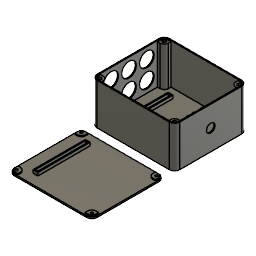
AC Box and Lid (Autodesk Fusion 360 design; units mm, degrees)
Autodesk Fusion 360 part; units mm, degrees
(part 1 of 2)
sketch "Sketch1" plane through (0, 0, 0) normal (0, 1, 0) x (1, 0, 0)
  line L0 (12.7, -101.6) -> (-165.1, -101.6)
  line L1 (-177.8, -88.9) -> (-177.8, 63.5)
  line L2 (-165.1, 76.2) -> (12.7, 76.2)
  line L3 (25.4, 63.5) -> (25.4, -88.9)
  arc A0 (-165.1, 76.2) -> (-177.8, 63.5) centre (-165.1, 63.5) ccw
  arc A1 (-177.8, -88.9) -> (-165.1, -101.6) centre (-165.1, -88.9) ccw
  arc A2 (25.4, 63.5) -> (12.7, 76.2) centre (12.7, 63.5) ccw
  arc A3 (12.7, -101.6) -> (25.4, -88.9) centre (12.7, -88.9) ccw
  line L4 (-158.75, 57.15) -> (-177.8, 57.15)
  line L5 (-177.8, 57.15) -> (-177.8, 76.2)
  line L6 (-177.8, 76.2) -> (-158.75, 76.2)
  line L7 (-158.75, 76.2) -> (-158.75, 57.15)
  line L8 (-164.275, 68.9844) -> (-168.275, 71.2938)
  line L9 (-168.275, 71.2938) -> (-172.275, 68.9844)
  line L10 (-172.275, 68.9844) -> (-172.275, 64.3656)
  line L11 (-172.275, 64.3656) -> (-168.275, 62.0562)
  line L12 (-168.275, 62.0562) -> (-164.275, 64.3656)
  line L13 (-164.275, 64.3656) -> (-164.275, 68.9844)
  line L14 (6.35, 76.2) -> (25.4, 76.2)
  line L15 (25.4, 57.15) -> (6.35, 57.15)
  line L16 (11.875, 68.9844) -> (11.875, 64.3656)
  line L17 (19.875, 64.3656) -> (19.875, 68.9844)
  line L18 (25.4, 76.2) -> (25.4, 57.15)
  line L19 (19.875, 68.9844) -> (15.875, 71.2938)
  line L20 (15.875, 71.2938) -> (11.875, 68.9844)
  line L21 (11.875, 64.3656) -> (15.875, 62.0562)
  line L22 (15.875, 62.0562) -> (19.875, 64.3656)
  line L23 (6.35, 57.15) -> (6.35, 76.2)
  line L24 (-177.8, -82.55) -> (-158.75, -82.55)
  line L25 (-158.75, -101.6) -> (-177.8, -101.6)
  line L26 (-172.275, -89.7656) -> (-172.275, -94.3844)
  line L27 (-164.275, -94.3844) -> (-164.275, -89.7656)
  line L28 (-158.75, -82.55) -> (-158.75, -101.6)
  line L29 (-164.275, -89.7656) -> (-168.275, -87.4562)
  line L30 (-168.275, -87.4562) -> (-172.275, -89.7656)
  line L31 (-172.275, -94.3844) -> (-168.275, -96.6938)
  line L32 (-168.275, -96.6938) -> (-164.275, -94.3844)
  line L33 (-177.8, -101.6) -> (-177.8, -82.55)
  line L34 (6.35, -82.55) -> (25.4, -82.55)
  line L35 (25.4, -101.6) -> (6.35, -101.6)
  line L36 (11.875, -89.7656) -> (11.875, -94.3844)
  line L37 (19.875, -94.3844) -> (19.875, -89.7656)
  line L38 (25.4, -82.55) -> (25.4, -101.6)
  line L39 (19.875, -89.7656) -> (15.875, -87.4562)
  line L40 (15.875, -87.4562) -> (11.875, -89.7656)
  line L41 (11.875, -94.3844) -> (15.875, -96.6938)
  line L42 (15.875, -96.6938) -> (19.875, -94.3844)
  line L43 (6.35, -101.6) -> (6.35, -82.55)
  circle A4 centre (-168.275, 66.675) radius 3.175
  circle A5 centre (-168.275, -92.075) radius 3.175
  circle A6 centre (15.875, -92.075) radius 3.175
  circle A7 centre (15.875, 66.675) radius 3.175
  point P0 (0, -101.6)
  point P1 (-177.8, -101.6)
  point P2 (25.4, 76.2)
  point P3 (-168.275, 66.675)
  point P4 (-6.35, 76.2)
  point P5 (-19.05, 63.5)
  point P6 (-6.35, 63.5)
  point P7 (15.875, 66.675)
  point P8 (-165.1, -82.55)
  point P9 (-177.8, -19.05)
  point P10 (-165.1, -95.25)
  point P11 (-168.275, -92.075)
  point P12 (-6.35, -6.35)
  point P13 (-19.05, -19.05)
  point P14 (-6.35, -19.05)
  point P15 (15.875, -92.075)
  dimension "d1" = 177.8
  dimension "d3" = 12.7
  dimension "d4" = 12.7
  dimension "d5" = 12.7
  dimension "d6" = 12.7
  dimension "d7" = 4
  dimension "d12" = 6.35
  dimension "d13" = 6.35
  dimension "d14" = 6.35
  dimension "d15" = 6.35
  dimension "d138" = 203.2
  dimension "d195" = 152.4
  constraint vertical L1
  constraint horizontal L2
  constraint vertical L3
  constraint tangent L1 A0
  constraint tangent L2 A0
  constraint coincident P1 L1
  constraint coincident P1 L0
  constraint tangent L1 A1
  constraint tangent L0 A1
  constraint coincident P2 L2
  constraint coincident P2 L3
  constraint tangent L2 A2
  constraint tangent L3 A2
  constraint tangent L3 A3
  constraint tangent L0 A3
  constraint horizontal L4
  constraint vertical L5
  constraint horizontal L6
  constraint vertical L7
  constraint coincident P3 A4.centre
  constraint coincident P11 A5.centre
  constraint coincident P15 A6.centre
  constraint coincident P7 A7.centre
  measures "d1" distance of P0 L25.end
  measures "d3" radius of A0
  measures "d4" radius of A1
  measures "d5" radius of A2
  measures "d6" radius of A3
  measures "d7" distance of P3 L13
  measures "d12" diameter of A4
  measures "d13" diameter of A5
  measures "d14" diameter of A6
  measures "d15" diameter of A7
  measures "d138" distance of L1 L3
  measures "d195" distance of L1.end L1.start
  measures "d385" diameter of L27.end
extrude "Extrude1" add sketch "Sketch1" along normal blind 101.6 contours L0 L3 A3 L34 L35 L38 L43 | L0 L1 L2 L3 L4 L7 L15 L23 L24 L28 L34 L43 | L0 L1 A1 L24 L25 L28 L33 | L2 L3 A2 L14 L15 L18 L23 | L1 L2 A0 L4 L5 L6 L7 | L8 L9 L10 L11 L12 L13 | L16 L17 L19 L20 L21 L22 | L26 L27 L29 L30 L31 L32 | L36 L37 L39 L40 L41 L42 | A4 | A5 | A6 | A7 makes body 1
shell "Shell1" thickness 2.54 removed faces 1 at (-103.7167, 101.6, -16.9333) on bodies 1
extrude "Extrude2" add sketch "Sketch1" along normal blind 99.06 contours L0 L3 A3 L34 L35 L38 L43 | L0 L1 A1 L24 L25 L28 L33 | L2 L3 A2 L14 L15 L18 L23 | L1 L2 A0 L4 L5 L6 L7 bodies 1
extrude "Extrude3" add sketch "Sketch1" along normal blind 93.98 contours L8 L9 L10 L11 L12 L13 | L16 L17 L19 L20 L21 L22 | L26 L27 L29 L30 L31 L32 | L36 L37 L39 L40 L41 L42 bodies 1
fillet "Fillet1" radius 10.16 4 edges at (-158.75, 50.8, -57.15) (-158.75, 50.8, 82.55) (6.35, 50.8, -57.15) (6.35, 50.8, 82.55) on bodies 1
sketch "Sketch3" plane through (0, 0, 0) normal (0, 1, 0) x (1, 0, 0)
  line L0 (-165.1, -127) -> (12.7, -127)
  line L1 (25.4, -139.7) -> (25.4, -292.1)
  line L2 (12.7, -304.8) -> (-165.1, -304.8)
  line L3 (-177.8, -292.1) -> (-177.8, -139.7)
  arc A0 (-165.1, -127) -> (-177.8, -139.7) centre (-165.1, -139.7) ccw
  arc A1 (25.4, -139.7) -> (12.7, -127) centre (12.7, -139.7) ccw
  arc A2 (-177.8, -292.1) -> (-165.1, -304.8) centre (-165.1, -292.1) ccw
  arc A3 (12.7, -304.8) -> (25.4, -292.1) centre (12.7, -292.1) ccw
  line L4 (-168.91, -146.05) -> (-177.8, -146.05)
  line L5 (-177.8, -146.05) -> (-177.8, -127)
  line L6 (-177.8, -127) -> (-158.75, -127)
  line L7 (-158.75, -127) -> (-158.75, -135.89)
  circle A4 centre (-168.275, -136.525) radius 3
  line L8 (25.4, -285.75) -> (16.51, -285.75)
  line L9 (6.35, -295.91) -> (6.35, -304.8)
  line L10 (6.35, -304.8) -> (25.4, -304.8)
  line L11 (25.4, -304.8) -> (25.4, -285.75)
  circle A5 centre (15.875, -295.275) radius 3
  circle A6 centre (15.875, -136.525) radius 3
  circle A7 centre (-168.275, -295.275) radius 3
  line L12 (-177.8, -304.8) -> (-158.75, -304.8)
  line L13 (-158.75, -304.8) -> (-158.75, -295.91)
  line L14 (-168.91, -285.75) -> (-177.8, -285.75)
  line L15 (-177.8, -285.75) -> (-177.8, -304.8)
  line L16 (16.51, -146.05) -> (25.4, -146.05)
  line L17 (25.4, -146.05) -> (25.4, -127)
  line L18 (25.4, -127) -> (6.35, -127)
  line L19 (6.35, -127) -> (6.35, -135.89)
  arc A8 (-168.91, -146.05) -> (-158.75, -135.89) centre (-168.91, -135.89) ccw
  arc A9 (-158.75, -295.91) -> (-168.91, -285.75) centre (-168.91, -295.91) ccw
  arc A10 (6.35, -135.89) -> (16.51, -146.05) centre (16.51, -135.89) ccw
  arc A11 (16.51, -285.75) -> (6.35, -295.91) centre (16.51, -295.91) ccw
  arc A12 (-165.1, -129.54) -> (-175.26, -139.7) centre (-165.1, -139.7) ccw
  line L20 (-175.26, -292.1) -> (-175.26, -139.7)
  arc A13 (-175.26, -292.1) -> (-165.1, -302.26) centre (-165.1, -292.1) ccw
  line L21 (12.7, -302.26) -> (-165.1, -302.26)
  arc A14 (12.7, -302.26) -> (22.86, -292.1) centre (12.7, -292.1) ccw
  line L22 (22.86, -139.7) -> (22.86, -292.1)
  arc A15 (22.86, -139.7) -> (12.7, -129.54) centre (12.7, -139.7) ccw
  line L23 (-165.1, -129.54) -> (12.7, -129.54)
  line L24 (6.35, -129.54) -> (3.81, -129.54)
  circle A16 centre (-168.275, -136.525) radius 5
  circle A17 centre (-168.275, -295.275) radius 5
  circle A18 centre (15.875, -295.275) radius 5
  circle A19 centre (15.875, -136.525) radius 5
  dimension "d28" = 12.7
  dimension "d29" = 12.7
  dimension "d30" = 12.7
  dimension "d31" = 12.7
  dimension "d32" = 6
  dimension "d34" = 6
  dimension "d35" = 6
  dimension "d36" = 6
  dimension "d39" = 19.05
  dimension "d40" = 10.16
  dimension "d41" = 10.16
  dimension "d42" = 10.16
  dimension "d43" = 10.16
  dimension "d44" = 2.54
  dimension "d68" = 10
  dimension "d69" = 10
  dimension "d70" = 10
  dimension "d71" = 10
  dimension "d139" = 198.12
  dimension "d196" = 152.4
  constraint horizontal L0
  constraint vertical L1
  constraint horizontal L2
  constraint vertical L3
  constraint tangent L0 A0
  constraint tangent L3 A0
  constraint tangent L0 A1
  constraint tangent L1 A1
  constraint tangent L3 A2
  constraint tangent L2 A2
  constraint tangent L1 A3
  constraint tangent L2 A3
  constraint horizontal L4
  constraint vertical L5
  constraint horizontal L6
  constraint vertical L7
  constraint horizontal L8
  constraint vertical L9
  constraint horizontal L10
  constraint vertical L11
  constraint horizontal L12
  constraint vertical L13
  constraint horizontal L14
  constraint vertical L15
  constraint horizontal L16
  constraint vertical L17
  constraint horizontal L18
  constraint vertical L19
  constraint tangent L4 A8
  constraint tangent L7 A8
  constraint tangent L13 A9
  constraint tangent L14 A9
  constraint tangent L16 A10
  constraint tangent L19 A10
  constraint tangent L8 A11
  constraint tangent L9 A11
  constraint horizontal L24
  constraint coincident L23 L24.start
  constraint coincident L19 L24.start
  constraint concentric A4 A16
  constraint concentric A7 A17
  constraint concentric A5 A18
  constraint concentric A6 A19
  measures "d28" radius of A0
  measures "d29" radius of A1
  measures "d30" radius of A2
  measures "d31" radius of A3
  measures "d32" diameter of A4
  measures "d34" diameter of A5
  measures "d35" diameter of A6
  measures "d36" diameter of A7
  measures "d39" distance of L12.start L14.end
  measures "d40" radius of A8
  measures "d41" radius of A9
  measures "d42" radius of A10
  measures "d43" radius of A11
  measures "d68" diameter of A16
  measures "d69" diameter of A17
  measures "d70" diameter of A18
  measures "d71" diameter of A19
  measures "d139" distance of L20 L22
  measures "d196" distance of L3.end L3.start
extrude "Extrude5" add sketch "Sketch3" along normal blind 3.81 separate body contours L0 L3 A0 L4 L5 L6 L7 A12 L20 L23 | L0 L7 L19 L23 L24 | L0 L1 A1 L16 L17 L18 L19 L22 A15 L23 | L4 L7 L8 L9 L13 L14 L16 L19 A8 A9 A10 A11 L20 L21 L22 L23 L24 | L4 L7 A8 A12 L20 L23 | L3 L4 L14 L20 | L16 L19 A10 L22 A15 L23 | L2 L3 A2 L12 L13 L14 L15 L20 A13 L21 | L13 L14 A9 L20 A13 L21 | L1 L8 L16 L22 | L1 L2 A3 L8 L9 L10 L11 L21 A14 L22 | L2 L9 L13 L21 | L8 L9 A11 L21 A14 L22 | A16 | A17 | A18 | A19 makes body 2
extrude "Extrude6" add sketch "Sketch3" along normal blind 6.35 contours L4 L7 A8 A12 L20 L23 | L16 L19 A10 L22 A15 L23 | L13 L14 A9 L20 A13 L21 | L8 L9 A11 L21 A14 L22 | A16 | A17 | A18 | A19 bodies 2
chamfer "Chamfer1" distance 2.032 angle 45 4 edges at (13.078, 0, 135.4402) (13.078, 0, 294.1902) (-171.072, 0, 135.4402) (-171.072, 0, 294.1902) on bodies 2
sketch "Sketch10" plane through (-175.26, 0, 0) normal (1, 0, 0) x (0, 0, -1)
  line L0 (57.15, 2.54) -> (57.15, 99.06)
  line L1 (57.15, 99.06) -> (63.5, 99.06)
  line L2 (63.5, 99.06) -> (63.5, 101.6)
  line L3 (63.5, 101.6) -> (-88.9, 101.6)
  line L4 (-88.9, 101.6) -> (-88.9, 99.06)
  line L5 (-88.9, 99.06) -> (-82.55, 99.06)
  line L6 (-82.55, 99.06) -> (-82.55, 2.54)
  line L7 (-82.55, 2.54) -> (57.15, 2.54)
  line L8 (-82.55, 2.54) -> (-82.55, 101.6) construction
  line L9 (-82.55, 101.6) -> (-74.2569, 101.6) construction
  line L10 (-74.2569, 101.6) -> (-74.2569, 92.2528) construction
  line L11 (-74.2569, 92.2528) -> (-82.55, 92.2528) construction
  line L12 (-82.55, 92.2528) -> (-82.55, 101.6) construction
  line L13 (57.15, 101.6) -> (31.1023, 101.6) construction
  line L14 (31.1023, 101.6) -> (31.1023, 74.4982) construction
  line L15 (31.1023, 74.4982) -> (57.15, 74.4982) construction
  line L16 (57.15, 74.4982) -> (57.15, 101.6) construction
  circle A0 centre (31.1023, 74.4982) radius 17.7546
  line L17 (-82.55, 101.6) -> (-56.5023, 101.6) construction
  line L18 (-56.5023, 101.6) -> (-56.5023, 74.4982) construction
  line L19 (-56.5023, 74.4982) -> (-82.55, 74.4982) construction
  line L20 (-82.55, 74.4982) -> (-82.55, 101.6) construction
  line L21 (-56.5023, 2.54) -> (-56.5023, 29.6418) construction
  line L22 (-56.5023, 74.4982) -> (31.1023, 74.4982) construction
  circle A1 centre (-12.7, 74.4982) radius 17.7546
  circle A2 centre (-56.5023, 74.4982) radius 17.7546
  circle A3 centre (31.1023, 29.6418) radius 17.7546
  circle A4 centre (-12.7, 29.6418) radius 17.7546
  circle A5 centre (-56.5023, 29.6418) radius 17.7546
  line L23 (-38.7477, 74.4982) -> (-38.7477, 2.54) construction
  line L24 (-74.2569, 74.4982) -> (-74.2569, 2.54) construction
  line L25 (-30.4546, 74.4982) -> (-30.4546, 2.54) construction
  line L26 (5.0546, 74.4982) -> (5.0546, 2.54) construction
  line L27 (13.3477, 74.4982) -> (13.3477, 2.54) construction
  line L28 (48.8569, 74.4982) -> (48.8569, 2.54) construction
  line L29 (-39.0023, 91.9982) -> (-39.0023, 56.9982)
  line L30 (-56.5023, 74.4982) -> (-39.0023, 74.4982) construction
  line L31 (-56.5023, 91.9982) -> (-56.5023, 56.9982) construction
  circle A6 centre (-50.7316, 77.9802) radius 3.7
  circle A7 centre (-62.3334, 77.8956) radius 3.7
  line L32 (-39.0023, 74.4982) -> (-39.0023, 91.9982) construction
  line L33 (-39.0023, 56.9982) -> (-74.0023, 56.9982)
  circle A8 centre (-50.3617, 86.7403) radius 1.25
  line L34 (-39.0023, 56.9982) -> (-39.0023, 91.9982) construction
  circle A9 centre (-56.5023, 74.4982) radius 17.5
  circle A10 centre (-65.2414, 63.5652) radius 1.25
  circle A11 centre (-59.9313, 63.1667) radius 3
  line L35 (-74.0023, 91.9982) -> (-39.0023, 91.9982)
  line L36 (-74.0023, 74.4982) -> (-39.0023, 74.4982) construction
  line L37 (-74.0023, 56.9982) -> (-74.0023, 91.9982)
  line L38 (-39.0023, 91.9982) -> (-56.5023, 91.9982) construction
  line L39 (-56.5023, 91.9982) -> (-56.5023, 74.4982) construction
  line L40 (4.8, 91.9982) -> (4.8, 56.9982)
  line L41 (-12.7, 74.4982) -> (4.8, 74.4982) construction
  line L42 (-12.7, 91.9982) -> (-12.7, 56.9982) construction
  circle A12 centre (-6.9293, 77.9802) radius 3.7
  circle A13 centre (-18.5311, 77.8956) radius 3.7
  line L43 (4.8, 74.4982) -> (4.8, 91.9982) construction
  line L44 (4.8, 56.9982) -> (-30.2, 56.9982)
  circle A14 centre (-6.5594, 86.7403) radius 1.25
  line L45 (4.8, 56.9982) -> (4.8, 91.9982) construction
  circle A15 centre (-12.7, 74.4982) radius 17.5
  circle A16 centre (-21.4391, 63.5652) radius 1.25
  circle A17 centre (-16.129, 63.1667) radius 3
  line L46 (-30.2, 91.9982) -> (4.8, 91.9982)
  line L47 (-30.2, 74.4982) -> (4.8, 74.4982) construction
  line L48 (-30.2, 56.9982) -> (-30.2, 91.9982)
  line L49 (4.8, 91.9982) -> (-12.7, 91.9982) construction
  line L50 (-12.7, 91.9982) -> (-12.7, 74.4982) construction
  line L51 (-74.0023, 29.6418) -> (-39.0023, 29.6418) construction
  line L52 (-56.5023, 29.6418) -> (-39.0023, 29.6418) construction
  circle A18 centre (-56.5023, 29.6418) radius 17.5
  line L53 (-39.0023, 29.6418) -> (-39.0023, 47.1418) construction
  circle A19 centre (-65.2414, 18.7088) radius 1.25
  line L54 (-56.5023, 47.1418) -> (-56.5023, 29.6418) construction
  line L55 (-39.0023, 47.1418) -> (-39.0023, 12.1418)
  circle A20 centre (-50.3617, 41.8839) radius 1.25
  line L56 (-39.0023, 12.1418) -> (-74.0023, 12.1418)
  line L57 (-74.0023, 12.1418) -> (-74.0023, 47.1418)
  circle A21 centre (-59.9313, 18.3103) radius 3
  line L58 (-39.0023, 47.1418) -> (-56.5023, 47.1418) construction
  line L59 (-74.0023, 47.1418) -> (-39.0023, 47.1418)
  line L60 (-56.5023, 47.1418) -> (-56.5023, 12.1418) construction
  circle A22 centre (-50.7316, 33.1238) radius 3.7
  circle A23 centre (-62.3334, 33.0392) radius 3.7
  line L61 (-39.0023, 12.1418) -> (-39.0023, 47.1418) construction
  line L62 (-30.2, 29.6418) -> (4.8, 29.6418) construction
  line L63 (-30.2, 47.1418) -> (4.8, 47.1418)
  circle A24 centre (-12.7, 29.6418) radius 17.5
  line L64 (-12.7, 29.6418) -> (4.8, 29.6418) construction
  circle A25 centre (-16.129, 18.3103) radius 3
  line L65 (4.8, 47.1418) -> (-12.7, 47.1418) construction
  line L66 (-12.7, 47.1418) -> (-12.7, 29.6418) construction
  circle A26 centre (-18.5311, 33.0392) radius 3.7
  line L67 (4.8, 47.1418) -> (4.8, 12.1418)
  line L68 (-12.7, 47.1418) -> (-12.7, 12.1418) construction
  line L69 (4.8, 29.6418) -> (4.8, 47.1418) construction
  line L70 (4.8, 12.1418) -> (4.8, 47.1418) construction
  circle A27 centre (-6.5594, 41.8839) radius 1.25
  line L71 (4.8, 12.1418) -> (-30.2, 12.1418)
  circle A28 centre (-6.9293, 33.1238) radius 3.7
  circle A29 centre (-21.4391, 18.7088) radius 1.25
  line L72 (-30.2, 12.1418) -> (-30.2, 47.1418)
  line L73 (13.6023, 29.6418) -> (48.6023, 29.6418) construction
  line L74 (13.6023, 47.1418) -> (48.6023, 47.1418)
  circle A30 centre (31.1023, 29.6418) radius 17.5
  line L75 (31.1023, 29.6418) -> (48.6023, 29.6418) construction
  circle A31 centre (27.6733, 18.3103) radius 3
  line L76 (48.6023, 47.1418) -> (31.1023, 47.1418) construction
  line L77 (31.1023, 47.1418) -> (31.1023, 29.6418) construction
  circle A32 centre (25.2712, 33.0392) radius 3.7
  line L78 (48.6023, 47.1418) -> (48.6023, 12.1418)
  line L79 (31.1023, 47.1418) -> (31.1023, 12.1418) construction
  line L80 (48.6023, 29.6418) -> (48.6023, 47.1418) construction
  line L81 (48.6023, 12.1418) -> (48.6023, 47.1418) construction
  circle A33 centre (37.2429, 41.8839) radius 1.25
  line L82 (48.6023, 12.1418) -> (13.6023, 12.1418)
  circle A34 centre (36.873, 33.1238) radius 3.7
  circle A35 centre (22.3632, 18.7088) radius 1.25
  line L83 (13.6023, 12.1418) -> (13.6023, 47.1418)
  line L84 (13.6023, 74.4982) -> (48.6023, 74.4982) construction
  line L85 (13.6023, 91.9982) -> (48.6023, 91.9982)
  circle A36 centre (31.1023, 74.4982) radius 17.5
  line L86 (31.1023, 74.4982) -> (48.6023, 74.4982) construction
  circle A37 centre (27.6733, 63.1667) radius 3
  line L87 (48.6023, 91.9982) -> (31.1023, 91.9982) construction
  line L88 (31.1023, 91.9982) -> (31.1023, 74.4982) construction
  circle A38 centre (25.2712, 77.8956) radius 3.7
  line L89 (48.6023, 91.9982) -> (48.6023, 56.9982)
  line L90 (31.1023, 91.9982) -> (31.1023, 56.9982) construction
  line L91 (48.6023, 74.4982) -> (48.6023, 91.9982) construction
  line L92 (48.6023, 56.9982) -> (48.6023, 91.9982) construction
  circle A39 centre (37.2429, 86.7403) radius 1.25
  line L93 (48.6023, 56.9982) -> (13.6023, 56.9982)
  circle A40 centre (36.873, 77.9802) radius 3.7
  circle A41 centre (22.3632, 63.5652) radius 1.25
  line L94 (13.6023, 56.9982) -> (13.6023, 91.9982)
  line L95 (-74.0023, 91.9982) -> (-74.0161, 101.6) construction
  line L96 (-74.0161, 101.6) -> (48.6023, 101.6)
  line L97 (48.6023, 101.6) -> (48.6023, 2.54)
  line L98 (48.6023, 2.54) -> (-74.0161, 2.54)
  line L99 (-74.0161, 2.54) -> (-74.0161, 101.6)
  point P0 (-56.5023, 131.8455)
  point P1 (-56.5023, 74.4982)
  point P2 (-50.3617, 86.7403)
  point P3 (-56.5023, 131.8455)
  point P4 (-12.7, 154.7055)
  point P5 (-12.7, 74.4982)
  point P6 (-6.5594, 86.7403)
  point P7 (9.303, 164.289)
  point P8 (-12.7, 154.7055)
  point P9 (9.303, 164.289)
  point P10 (-50.3617, 41.8839)
  point P11 (-56.5023, 29.6418)
  point P12 (-56.5023, 154.7055)
  point P13 (-56.5023, 154.7055)
  point P14 (9.303, 164.289)
  point P15 (9.303, 164.289)
  point P16 (-12.7, 29.6418)
  point P17 (-12.7, 154.7055)
  point P18 (-6.5594, 41.8839)
  point P19 (-12.7, 154.7055)
  point P20 (9.303, 164.289)
  point P21 (9.303, 164.289)
  point P22 (31.1023, 29.6418)
  point P23 (31.1023, 154.7055)
  point P24 (37.2429, 41.8839)
  point P25 (31.1023, 154.7055)
  point P26 (9.303, 164.289)
  point P27 (9.303, 164.289)
  point P28 (31.1023, 74.4982)
  point P29 (31.1023, 154.7055)
  point P30 (37.2429, 86.7403)
  point P31 (31.1023, 154.7055)
  dimension "d199" = 8.2931
  dimension "d200" = 9.3472
  dimension "d201" = 26.0477
  dimension "d202" = 27.1018
  dimension "d203" = 35.5092
  dimension "d204" = 26.0477
  dimension "d205" = 27.1018
  dimension "d206" = 27.1018
  dimension "d207" = 87.6046
  dimension "d208" = 44.8564
  dimension "d211" = -87.6046
  dimension "d212" = -44.8564
  dimension "d271" = 2.5
  dimension "d272" = 35
  dimension "d273" = 2.5
  dimension "d274" = 7.4
  dimension "d275" = 7.4
  dimension "d276" = 6
  dimension "d277" = 12.2421
  dimension "d278" = 6.1406
  dimension "d279" = 5.7707
  dimension "d280" = 3.3974
  dimension "d281" = 5.8311
  dimension "d282" = 11.3315
  dimension "d283" = 3.482
  dimension "d284" = 8.7391
  dimension "d285" = 10.933
  dimension "d286" = 3.429
  dimension "d289" = 35
  dimension "d290" = 2.5
  dimension "d291" = 35
  dimension "d292" = 2.5
  dimension "d293" = 7.4
  dimension "d294" = 7.4
  dimension "d295" = 6
  dimension "d296" = 12.2421
  dimension "d297" = 6.1406
  dimension "d298" = 5.7707
  dimension "d299" = 3.3974
  dimension "d300" = 5.8311
  dimension "d301" = 11.3315
  dimension "d302" = 3.482
  dimension "d303" = 8.7391
  dimension "d304" = 10.933
  dimension "d305" = 3.429
  dimension "d306" = 35
  dimension "d307" = 2.5
  dimension "d308" = 35
  dimension "d309" = 2.5
  dimension "d310" = 7.4
  dimension "d311" = 7.4
  dimension "d312" = 6
  dimension "d313" = 12.2421
  dimension "d314" = 6.1406
  dimension "d315" = 5.7707
  dimension "d316" = 3.3974
  dimension "d317" = 5.8311
  dimension "d318" = 11.3315
  dimension "d319" = 3.482
  dimension "d320" = 8.7391
  dimension "d321" = 10.933
  dimension "d322" = 3.429
  dimension "d323" = 35
  dimension "d324" = 2.5
  dimension "d325" = 35
  dimension "d326" = 2.5
  dimension "d327" = 7.4
  dimension "d328" = 7.4
  dimension "d329" = 6
  dimension "d330" = 12.2421
  dimension "d331" = 6.1406
  dimension "d332" = 5.7707
  dimension "d333" = 3.3974
  dimension "d334" = 5.8311
  dimension "d335" = 11.3315
  dimension "d336" = 3.482
  dimension "d337" = 8.7391
  dimension "d338" = 10.933
  dimension "d339" = 3.429
  dimension "d340" = 35
  dimension "d341" = 2.5
  dimension "d342" = 35
  dimension "d343" = 2.5
  dimension "d344" = 7.4
  dimension "d345" = 7.4
  dimension "d346" = 6
  dimension "d347" = 12.2421
  dimension "d348" = 6.1406
  dimension "d349" = 5.7707
  dimension "d350" = 3.3974
  dimension "d351" = 5.8311
  dimension "d352" = 11.3315
  dimension "d353" = 3.482
  dimension "d354" = 8.7391
  dimension "d355" = 10.933
  dimension "d356" = 3.429
  dimension "d357" = 35
  dimension "d358" = 2.5
  dimension "d359" = 35
  dimension "d360" = 2.5
  dimension "d361" = 7.4
  dimension "d362" = 7.4
  dimension "d363" = 6
  dimension "d364" = 12.2421
  dimension "d365" = 6.1406
  dimension "d366" = 5.7707
  dimension "d367" = 3.3974
  dimension "d368" = 5.8311
  dimension "d369" = 11.3315
  dimension "d370" = 3.482
  dimension "d371" = 8.7391
  dimension "d372" = 10.933
  dimension "d373" = 3.429
  dimension "d374" = 35
  constraint coincident L6.end L7.start
  constraint coincident L3 L8.end
  constraint perpendicular L3 L8
  constraint horizontal L9
  constraint vertical L10
  constraint horizontal L11
  constraint vertical L12
  constraint horizontal L13
  constraint vertical L14
  constraint horizontal L15
  constraint vertical L16
  constraint coincident L3 L13.start
  constraint coincident P28 L14.end
  constraint horizontal L17
  constraint vertical L18
  constraint horizontal L19
  constraint vertical L20
  constraint coincident L7 L21.start
  constraint perpendicular L7 L21
  constraint coincident A2 L23.start
  constraint coincident L22 L23.start
  constraint coincident L7 L23.end
  constraint tangent A2 L23
  constraint coincident L19 L24.start
  constraint coincident A2 L24.start
  constraint coincident L7 L24.end
  constraint tangent A2 L24
  constraint coincident A1 L25.start
  constraint coincident L22 L25.start
  constraint coincident L7 L25.end
  constraint tangent A1 L25
  constraint coincident L22 L26.start
  constraint coincident A1 L26.start
  constraint coincident L7 L26.end
  constraint tangent A1 L26
  constraint coincident A0 L27.start
  constraint coincident L22 L27.start
  constraint coincident L7 L27.end
  constraint tangent A0 L27
  constraint coincident A0 L28.start
  constraint coincident L15 L28.start
  constraint coincident L7 L28.end
  constraint tangent A0 L28
  constraint coincident P2 A8.centre
  constraint midpoint P1 L36
  constraint coincident P1 L18.end
  constraint coincident L30.end A9
  constraint horizontal L36
  constraint perpendicular L30 L32
  constraint parallel L30 L38
  constraint parallel L32 L39
  constraint parallel L30 L36
  constraint midpoint L30.end L34
  constraint perpendicular L29 L33
  constraint parallel L29 L37
  constraint parallel L33 L35
  constraint midpoint L31.end L33
  constraint perpendicular L31 L33
  constraint coincident P3 L31
  constraint coincident P3 P0
  constraint coincident P6 A14.centre
  constraint midpoint P5 L47
  constraint coincident P5 A1.centre
  constraint coincident L41.end A15
  constraint horizontal L47
  constraint perpendicular L41 L43
  constraint parallel L41 L49
  constraint parallel L43 L50
  constraint parallel L41 L47
  constraint midpoint L41.end L45
  constraint perpendicular L40 L44
  constraint parallel L40 L48
  constraint parallel L44 L46
  constraint midpoint L42.end L44
  constraint perpendicular L42 L44
  constraint coincident P19 L42
  constraint coincident P19 P17
  constraint coincident P10 A20.centre
  constraint midpoint P11 L51
  constraint coincident P11 L21.end
  constraint coincident L51.end A18
  constraint horizontal L51
  constraint perpendicular L52 L53
  constraint parallel L52 L58
  constraint parallel L53 L54
  constraint parallel L51 L52
  constraint midpoint L51.end L61
  constraint perpendicular L55 L56
  constraint parallel L55 L57
  constraint parallel L56 L59
  constraint midpoint L60.end L56
  constraint perpendicular L56 L60
  constraint coincident P13 L60
  constraint coincident P13 P12
  constraint coincident P18 A27.centre
  constraint midpoint P16 L62
  constraint coincident P16 A4.centre
  constraint coincident L62.end A24
  constraint horizontal L62
  constraint perpendicular L64 L69
  constraint parallel L64 L65
  constraint parallel L66 L69
  constraint parallel L62 L64
  constraint midpoint L62.end L70
  constraint perpendicular L67 L71
  constraint parallel L67 L72
  constraint parallel L63 L71
  constraint midpoint L68.end L71
  constraint perpendicular L68 L71
  constraint coincident P19 L68
  constraint coincident P24 A33.centre
  constraint midpoint P22 L73
  constraint coincident P22 A3.centre
  constraint coincident L73.end A30
  constraint horizontal L73
  constraint perpendicular L75 L80
  constraint parallel L75 L76
  constraint parallel L77 L80
  constraint parallel L73 L75
  constraint midpoint L73.end L81
  constraint perpendicular L78 L82
  constraint parallel L78 L83
  constraint parallel L74 L82
  constraint midpoint L79.end L82
  constraint perpendicular L79 L82
  constraint coincident P31 L79
  constraint coincident P31 P29
  constraint coincident P30 A39.centre
  constraint midpoint P28 L84
  constraint coincident L84.end A36
  constraint horizontal L84
  constraint perpendicular L86 L91
  constraint parallel L86 L87
  constraint parallel L88 L91
  constraint parallel L84 L86
  constraint midpoint L84.end L92
  constraint perpendicular L89 L93
  constraint parallel L89 L94
  constraint parallel L85 L93
  constraint midpoint L90.end L93
  constraint perpendicular L90 L93
  constraint coincident P31 L90
  constraint coincident L17 L95.end
  constraint horizontal L96
  constraint vertical L97
  constraint horizontal L98
  constraint vertical L99
  constraint coincident L7 L97.end
  measures "d199" distance of L8.end L9.end
  measures "d200" distance of L8.end L11.end
  measures "d201" distance of L13.start L13.end
  measures "d202" distance of L13.start L15.end
  measures "d203" diameter of A0
  measures "d204" distance of L8.end L17.end
  measures "d205" distance of L8.end L19.end
  measures "d206" distance of L21.start P11
  measures "d207" distance of P28 P1
  measures "d208" distance of P1 P11
  measures "d271" diameter of A8
  measures "d272" diameter of A9
  measures "d273" diameter of A10
  measures "d274" diameter of A6
  measures "d275" diameter of A7
  measures "d276" diameter of A11
  measures "d277" vertical distance of P2 P1
  measures "d278" horizontal distance of P2 P1
  measures "d279" horizontal distance of P1 A6.centre
  measures "d280" vertical distance of A7.centre P1
  measures "d281" horizontal distance of A7.centre P1
  measures "d282" vertical distance of A11.centre P1
  measures "d283" vertical distance of P1 A6.centre
  measures "d284" horizontal distance of A10.centre P1
  measures "d285" vertical distance of A10.centre P1
  measures "d286" horizontal distance of A11.centre P1
  measures "d289" distance of L29.start L29.end
  measures "d290" diameter of A14
  measures "d291" diameter of A15
  measures "d292" diameter of A16
  measures "d293" diameter of A12
  measures "d294" diameter of A13
  measures "d295" diameter of A17
  measures "d296" vertical distance of P6 P5
  measures "d297" horizontal distance of P6 P5
  measures "d298" horizontal distance of P5 A12.centre
  measures "d299" vertical distance of A13.centre P5
  measures "d300" horizontal distance of A13.centre P5
  measures "d301" vertical distance of A17.centre P5
  measures "d302" vertical distance of P5 A12.centre
  measures "d303" horizontal distance of A16.centre P5
  measures "d304" vertical distance of A16.centre P5
  measures "d305" horizontal distance of A17.centre P5
  measures "d306" distance of L40.start L40.end
  measures "d307" diameter of A20
  measures "d308" diameter of A18
  measures "d309" diameter of A19
  measures "d310" diameter of A22
  measures "d311" diameter of A23
  measures "d312" diameter of A21
  measures "d313" vertical distance of P11 P10
  measures "d314" horizontal distance of P11 P10
  measures "d315" horizontal distance of A22.centre P11
  measures "d316" vertical distance of A23.centre P11
  measures "d317" horizontal distance of A23.centre P11
  measures "d318" vertical distance of A21.centre P11
  measures "d319" vertical distance of A22.centre P11
  measures "d320" horizontal distance of A19.centre P11
  measures "d321" vertical distance of A19.centre P11
  measures "d322" horizontal distance of A21.centre P11
  measures "d323" distance of L53.end L55.end
  measures "d324" diameter of A27
  measures "d325" diameter of A24
  measures "d326" diameter of A29
  measures "d327" diameter of A28
  measures "d328" diameter of A26
  measures "d329" diameter of A25
  measures "d330" vertical distance of P16 P18
  measures "d331" horizontal distance of P16 P18
  measures "d332" horizontal distance of P16 A28.centre
  measures "d333" vertical distance of A26.centre P16
  measures "d334" horizontal distance of A26.centre P16
  measures "d335" vertical distance of A25.centre P16
  measures "d336" vertical distance of P16 A28.centre
  measures "d337" horizontal distance of A29.centre P16
  measures "d338" vertical distance of A29.centre P16
  measures "d339" horizontal distance of A25.centre P16
  measures "d340" distance of L63.end L67.end
  measures "d341" diameter of A33
  measures "d342" diameter of A30
  measures "d343" diameter of A35
  measures "d344" diameter of A34
  measures "d345" diameter of A32
  measures "d346" diameter of A31
  measures "d347" vertical distance of P22 P24
  measures "d348" horizontal distance of P22 P24
  measures "d349" horizontal distance of P22 A34.centre
  measures "d350" vertical distance of A32.centre P22
  measures "d351" horizontal distance of A32.centre P22
  measures "d352" vertical distance of A31.centre P22
  measures "d353" vertical distance of P22 A34.centre
  measures "d354" horizontal distance of A35.centre P22
  measures "d355" vertical distance of A35.centre P22
  measures "d356" horizontal distance of A31.centre P22
  measures "d357" distance of L74.end L78.end
  measures "d358" diameter of A39
  measures "d359" diameter of A36
  measures "d360" diameter of A41
  measures "d361" diameter of A40
  measures "d362" diameter of A38
  measures "d363" diameter of A37
  measures "d364" vertical distance of P28 P30
  measures "d365" horizontal distance of P28 P30
  measures "d366" horizontal distance of P28 A40.centre
  measures "d367" vertical distance of A38.centre P28
  measures "d368" horizontal distance of A38.centre P28
  measures "d369" vertical distance of A37.centre P28
  measures "d370" vertical distance of P28 A40.centre
  measures "d371" horizontal distance of A41.centre P28
  measures "d372" vertical distance of A41.centre P28
  measures "d373" horizontal distance of A37.centre P28
  measures "d374" distance of L85.end L89.end
sketch "Sketch11" plane through (0, 0, 0) normal (1, 0, 0) x (0, 1, 0)
  circle A0 centre (171.5579, 118.8164) radius 17.5
  line L0 (171.5579, 125.8164) -> (171.5579, 111.8164) construction
  line L1 (171.5579, 125.8164) -> (171.5579, 111.8164) construction
  line L2 (171.5579, 111.8164) -> (152.3803, 111.8164) construction
  line L3 (152.3803, 111.8164) -> (152.3803, 125.8164) construction
  line L4 (152.3803, 125.8164) -> (171.5579, 125.8164) construction
  line L5 (165.9188, 111.8164) -> (155.5188, 111.8164)
  line L6 (165.9188, 111.8164) -> (165.9188, 102.2498)
  line L7 (165.9188, 111.8164) -> (162.3188, 111.8164) construction
  line L8 (162.3188, 111.8164) -> (162.3188, 110.3164) construction
  line L9 (162.3188, 110.3164) -> (165.9188, 110.3164) construction
  line L10 (165.9188, 110.3164) -> (165.9188, 111.8164) construction
  line L11 (162.3188, 110.3164) -> (159.3188, 110.3164) construction
  circle A1 centre (160.8188, 110.3164) radius 1.5
  line L12 (165.9265, 125.8164) -> (165.9265, 135.3856)
  line L13 (165.9265, 125.8164) -> (155.5188, 125.8164)
  line L14 (160.8188, 110.3164) -> (160.8188, 108.8164) construction
  line L15 (171.5579, 118.8164) -> (154.0579, 118.8164) construction
  line L16 (154.0579, 118.8164) -> (179.9579, 118.8164) construction
  circle A2 centre (183.1575, 118.771) radius 3.2
  circle A3 centre (183.1575, 118.771) radius 3.95 construction
  circle A4 centre (184.8607, 125.7938) radius 1.55
  line L17 (171.5579, 118.8164) -> (171.5579, 136.3164) construction
  line L18 (171.5579, 136.3164) -> (188.9303, 136.3164) construction
  line L19 (185.223, 136.3164) -> (185.223, 124.3164) construction
  circle A5 centre (161.2232, 153.6549) radius 1.5
  circle A6 centre (185.2651, 169.1323) radius 1.55
  circle A7 centre (171.9623, 162.1549) radius 17.5
  point P0 (171.5579, 118.8164)
  dimension "d213" = 35
  dimension "d214" = 14
  dimension "d216" = 3.6
  dimension "d217" = 1.5
  dimension "d218" = 3
  dimension "d219" = 10.4
  dimension "d222" = 25.9
  dimension "d223" = 6.4
  dimension "d224" = 7.9
  dimension "d225" = 3.1
  dimension "d227" = 12
  dimension "d237" = 3.1
  dimension "d240" = 8.5
  dimension "d241" = 10.739
  dimension "d242" = 3
  dimension "d243" = 13.3028
  dimension "d244" = 6.9774
  dimension "d245" = 35
  constraint midpoint L0 P0
  constraint coincident P0 A0.centre
  constraint vertical L0
  constraint perpendicular L1 L2
  constraint parallel L1 L3
  constraint parallel L2 L4
  constraint coincident L2 L5.start
  constraint coincident A0 L5.end
  constraint coincident L2 L5.end
  constraint coincident A0 L6.end
  constraint perpendicular L5 L6
  constraint horizontal L7
  constraint vertical L8
  constraint horizontal L9
  constraint vertical L10
  constraint perpendicular L8 L11
  constraint coincident L11.end A1
  constraint coincident L8.end A1
  constraint coincident L4 L12.start
  constraint coincident A0 L12.end
  constraint perpendicular L4 L12
  constraint coincident A0 L13.end
  constraint coincident L4 L13.end
  constraint coincident A1.centre L14.start
  constraint coincident A1 L14.end
  constraint perpendicular L11 L14
  constraint coincident A0 L15.end
  constraint perpendicular L1 L15
  constraint perpendicular L0 L16
  constraint coincident L16.end A2
  constraint concentric A2 A3
  constraint coincident A0 L17.end
  constraint parallel L0 L17
  constraint tangent A0 L18
  constraint coincident L18 L19.start
  constraint perpendicular L18 L19
  measures "d213" diameter of A0
  measures "d214" distance of L0.start L0.end
  measures "d216" distance of L5.start L7.end
  measures "d217" distance of L5.start L9.end
  measures "d218" distance of L8.end L11.end
  measures "d219" distance of L5.start L5.end
  measures "d222" distance of L15.end L16.end
  measures "d223" diameter of A2
  measures "d224" diameter of A3
  measures "d225" diameter of A4
  measures "d227" distance of L19.start L19.end
  measures "d237" diameter of A6
  measures "d240" vertical distance of A5.centre A7.centre
  measures "d241" horizontal distance of A5.centre A7.centre
  measures "d242" diameter of A5
  measures "d243" horizontal distance of A6.centre A7.centre
  measures "d244" vertical distance of A6.centre A7.centre
  measures "d245" diameter of A7